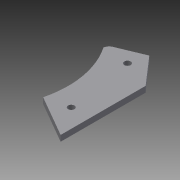
# Autodesk Inventor part: Eagle piece
Saved by Autodesk Inventor 2013 (Build 170138000, 138)
## iProperties
Created: 2014-05-22
Part Number: Eagle piece
Material: Generic
Document SubType Name: Modeling
Designer: kahohbein
Density: 1 g/cm^3
Author: kahohbein
Autodesk Inventor part; units mm, degrees
ref_plane "YZ Plane" through (0, 0, 0) normal (1, 0, 0) x (0, 1, 0)
ref_plane "XZ Plane" through (0, 0, 0) normal (0, 1, 0) x (-1, 0, 0)
ref_plane "XY Plane" through (0, 0, 0) normal (0, 0, 1) x (1, 0, 0)
sketch "Sketch1" plane through (0, 0, 0) normal (0, 1, 0) x (-1, 0, 0)
  line L0 (0, 0) -> (24.7467, -14.2875)
  line L1 (0, 0) -> (0, -50.8)
  line L2 (0, -50.8) -> (14.5809, -67.5734)
  arc A0 (29.2475, -61.4983) -> (32.4653, -58.0622) centre (28.1302, -57.2272) ccw
  arc A1 (24.7467, -14.2875) -> (32.4653, -58.0622) centre (77.3314, -27.5832) ccw
  line L3 (14.5809, -67.5734) -> (29.2475, -61.4983)
  circle A2 centre (17.1062, -57.0768) radius 1.905
  circle A3 centre (11.1033, -17.4625) radius 1.905
  line L4 (11.1033, -17.4625) -> (0, 0)
  line L5 (11.1033, -17.4625) -> (24.7467, -14.2875)
  line L6 (17.1062, -57.0768) -> (14.5809, -67.5734)
  line L7 (17.1062, -57.0768) -> (0, -50.8)
  dimension "d0" = 28.575
  dimension "d1" = 50.8
  dimension "d2" = 22.225
  dimension "d3" = 15.875
  dimension "d6" = 44.45
  dimension "d7" = 60
  dimension "d8" = 108.5
  dimension "d9" = 139
  dimension "d13" = 3.81
  dimension "d14" = 3.81
  dimension "d32" = 20.6935
  dimension "d33" = 17.1062
  dimension "d34" = 10.4967
  dimension "d35" = 13.6433
  constraints: 16 end point, 5 point on circle, 4 centre point, 1 coincident, 1 vertical
  measures "d0" distance of L0.start L0.end
  measures "d1" distance of L0.start L1.end
  measures "d2" distance of L1.end L2.end
  measures "d3" distance of L2.end L3.end
  measures "d6" distance of L0.end A0.end
  measures "d7" angle of L1 L0
  measures "d8" angle of L3 L2
  measures "d9" angle of L1 L2
  measures "d13" diameter of A2
  measures "d14" diameter of A3
  measures "d32" distance of L4.start L0.start
  measures "d33" horizontal distance of L6.start L1.end
  measures "d34" vertical distance of L6.start L2.end
  measures "d35" horizontal distance of L4.start L5.end
extrude "Extrusion1" add sketch "Sketch1" along normal blind 3.5052
sketch "Sketch2" plane through (0, 3.5052, 0) normal (0, 1, 0) x (1, 0, 0)
  circle A0 centre (-17.1062, 57.0768) radius 1.905
  circle A1 centre (-11.1033, 17.4625) radius 1.905
  dimension "d28" = 3.81
  dimension "d29" = 3.81
  constraints: 2 centre point
  measures "d28" diameter of A0
  measures "d29" diameter of A1
extrude "Extrusion2" cut sketch "Sketch2" against normal blind 3.5052
body "Solid1"
